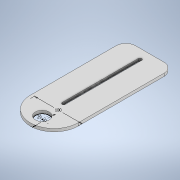
# Autodesk Inventor part: 零件1
Saved by Autodesk Inventor 2021 (Build 250183000, 183)
## iProperties
Created: 2022-06-11
Part Number: 零件1
Material: 一般
Document SubType Name: Modeling
Designer: 生活科技
Density: 1 g/cm^3
Appearance: 預設
Author: 生活科技
Autodesk Inventor part; units mm, degrees
ref_plane "YZ Plane" through (0, 0, 0) normal (1, 0, 0) x (0, 1, 0)
ref_plane "XZ Plane" through (0, 0, 0) normal (0, 1, 0) x (-1, 0, 0)
ref_plane "XY Plane" through (0, 0, 0) normal (0, 0, 1) x (1, 0, 0)
sketch "草圖1" plane through (0, 0, 0) normal (0, 1, 0) x (-1, 0, 0)
  line L0 (-100, 0) -> (-100, -180)
  line L1 (-80, -200) -> (-20, -200)
  line L2 (0, -180) -> (0, 0)
  arc A0 (0, 0) -> (-100, 0) centre (-50, 0) ccw
  arc A1 (-20, -200) -> (0, -180) centre (-20, -180) ccw
  arc A2 (-100, -180) -> (-80, -200) centre (-80, -180) ccw
  line L3 (-50, -180) -> (-50, -20) construction
  line L4 (-46.5, -180) -> (-46.5, -20)
  line L5 (-53.5, -20) -> (-53.5, -180)
  arc A3 (-53.5, -180) -> (-46.5, -180) centre (-50, -180) ccw
  arc A4 (-46.5, -20) -> (-53.5, -20) centre (-50, -20) ccw
  line L6 (-50, -180) -> (110, -180) construction
  line L7 (0, 0) -> (-100, 0) construction
  line L8 (-50, 0) -> (-50, 50) construction
  circle A5 centre (-50, 25) radius 14.5
  point P0 (-50, -100)
  dimension "d5" = 20
  dimension "d6" = 160
  dimension "d7" = 90
  dimension "d8" = 7
  dimension "d12" = 29
  constraints: 20 end point, 11 point on circle, 8 tangent, 6 centre point, 2 horizontal, 2 midpoint, 2 parallel, 1 equal radius, 1 perpendicular, 1 vertical
  measures "d5" radius of A1
  measures "d6" distance of L3.start L3.end
  measures "d7" angle of L6 L3
  measures "d8" diameter of A4
  measures "d12" diameter of A5
sketch "草圖2" plane through (0, 0, 0) normal (0, 1, 0) x (-1, 0, 0)
  line L0 (0, 0) -> (-100, 0)
  line L1 (-50, 0) -> (-50, 50) construction
  circle A0 centre (-50, 25) radius 14.5
  dimension "d9" = 100
  dimension "d10" = 50
  dimension "d11" = 29
  constraints: 4 end point, 2 midpoint, 1 centre point, 1 horizontal, 1 vertical
  measures "d9" distance of L0.start L0.end
  measures "d10" distance of L1.start L1.end
  measures "d11" diameter of A0
extrude "擠出1" add sketch "草圖1" along normal blind 6
